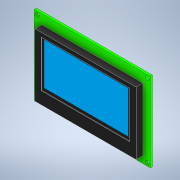
# Autodesk Inventor part: Adafruit_2675
Saved by Autodesk Inventor 2021 (Build 250183000, 183)
## iProperties
Created: 2020-11-05
Part Number: Adafruit_2675
Material: Generic
Document SubType Name: Modeling
Designer: Viktor
Density: 1 g/cm^3
Appearance: Default
Author: Viktor
Autodesk Inventor part; units mm, degrees
ref_plane "YZ Plane" through (0, 0, 0) normal (1, 0, 0) x (0, 1, 0)
ref_plane "XZ Plane" through (0, 0, 0) normal (0, 1, 0) x (-1, 0, 0)
ref_plane "XY Plane" through (0, 0, 0) normal (0, 0, 1) x (1, 0, 0)
sketch "Sketch1" plane through (0, 0, 0) normal (0, 0, 1) x (1, 0, 0)
  line L0 (-42.5, -29) -> (42.5, -29)
  line L1 (42.5, -29) -> (42.5, 29)
  line L2 (42.5, 29) -> (-42.5, 29)
  line L3 (-42.5, 29) -> (-42.5, -29)
  line L4 (-42.5, -29) -> (42.5, 29) construction
  line L5 (42.5, -29) -> (-42.5, 29) construction
  point P0 (0, 0)
  dimension "d0" = 85
  dimension "d1" = 58
  constraints: 12 end point, 2 midpoint, 2 parallel, 1 horizontal, 1 perpendicular
  measures "d0" distance of L1.end L2.end
  measures "d1" distance of L0.end L1.end
extrude "Extrusion1" add sketch "Sketch1" along normal blind 1.6
sketch "Sketch2" plane through (0, 0, 1.6) normal (0, 0, 1) x (1, 0, 0)
  line L0 (-59.5, 0) -> (59.5, 0) construction
  line L1 (0, -40.6) -> (0, 40.6) construction
  circle A0 centre (-40.3, 26.8) radius 1.6
  line L2 (42.5, 29) -> (-42.5, 29) construction
  line L3 (-42.5, 29) -> (-42.5, -29) construction
  circle A1 centre (40.3, 26.8) radius 1.6
  circle A2 centre (-40.3, -26.8) radius 1.6
  line L4 (42.5, -29) -> (-42.5, -29) construction
  circle A3 centre (40.3, -26.8) radius 1.6
  point P0 (0, 0)
  dimension "d4" = 3.2
  dimension "d5" = 0.6
  dimension "d6" = 0.6
  constraints: 4 centre point, 4 symmetric about line, 2 end point, 3 other
  measures "d4" diameter of A0
  measures "d5" distance edge to line of A0 L2
  measures "d6" distance edge to line of A0 L3
extrude "Extrusion2" cut sketch "Sketch2" against normal through all
sketch "Sketch3" plane through (0, 0, 1.6) normal (0, 0, 1) x (1, 0, 0)
  line L0 (0, 40.6) -> (0, -40.6) projected
  line L1 (-37, -24) -> (37, -24)
  line L2 (37, -24) -> (37, 22)
  line L3 (37, 22) -> (-37, 22)
  line L4 (-37, 22) -> (-37, -24)
  line L5 (-37, -24) -> (37, 22) construction
  line L6 (37, -24) -> (-37, 22) construction
  line L7 (-59.5, 0) -> (59.5, 0) projected
  point P0 (0, -1)
  dimension "d9" = 46
  dimension "d10" = 74
  dimension "d25" = 1
  constraints: 12 end point, 2 midpoint, 2 parallel, 1 horizontal, 1 perpendicular, 1 point on line
  measures "d9" distance of L3.end L1.start
  measures "d10" distance of L2.end L3.end
  measures "d25" distance from line of L7 point (0, -1)
extrude "Extrusion3" add sketch "Sketch3" along normal blind 5 separate body
sketch "Sketch4" plane through (0, 0, 6.6) normal (0, 0, 1) x (1, 0, 0)
  line L0 (0, -40.6) -> (0, 40.6) projected
  line L1 (-32.5, -15) -> (32.5, -15)
  line L2 (32.5, -15) -> (32.5, 19)
  line L3 (32.5, 19) -> (-32.5, 19)
  line L4 (-32.5, 19) -> (-32.5, -15)
  line L5 (-32.5, -15) -> (32.5, 19) construction
  line L6 (32.5, -15) -> (-32.5, 19) construction
  line L7 (37, 22) -> (-37, 22) projected
  point P0 (0, 0)
  point P1 (0, 2)
  dimension "d13" = 34
  dimension "d14" = 65
  dimension "d15" = 3
  constraints: 12 end point, 2 midpoint, 2 parallel, 1 horizontal, 1 perpendicular, 1 point on line
  measures "d13" distance of L3.end L1.start
  measures "d14" distance of L2.end L3.end
  measures "d15" distance between parallel lines of L7 L3
extrude "Extrusion4" cut sketch "Sketch4" against normal blind 0.5 bodies 2
sketch "Sketch5" plane through (0, 0, 6.1) normal (0, 0, 1) x (1, 0, 0)
  line L0 (0, 40.6) -> (0, -40.6) projected
  line L1 (-30.705, -12.69) -> (30.705, -12.69)
  line L2 (30.705, -12.69) -> (30.705, 18)
  line L3 (30.705, 18) -> (-30.705, 18)
  line L4 (-30.705, 18) -> (-30.705, -12.69)
  line L5 (-30.705, -12.69) -> (30.705, 18) construction
  line L6 (30.705, -12.69) -> (-30.705, 18) construction
  line L7 (37, 22) -> (-37, 22) projected
  point P0 (0, 0)
  point P1 (0, 2.655)
  dimension "d18" = 30.69
  dimension "d19" = 61.41
  dimension "d20" = 4
  constraints: 12 end point, 2 midpoint, 2 parallel, 1 horizontal, 1 perpendicular, 1 point on line
  measures "d18" distance of L3.end L1.start
  measures "d19" distance of L2.end L3.end
  measures "d20" distance between parallel lines of L7 L3
extrude "Extrusion5" cut sketch "Sketch5" against normal blind 0.5 bodies 2
sketch "Sketch6" plane through (0, 0, 5.6) normal (0, 0, 1) x (1, 0, 0)
  line L0 (30.705, -12.69) -> (-30.705, -12.69) projected
  line L1 (30.705, 18) -> (30.705, -12.69) projected
  line L2 (-30.705, 18) -> (30.705, 18) projected
  line L3 (-30.705, -12.69) -> (-30.705, 18) projected
  point P0 (0, 0)
extrude "Extrusion6" add sketch "Sketch6" along normal blind 0.5 separate body
sketch "Sketch7" plane through (0, 0, 6.6) normal (0, 0, 1) x (1, 0, 0)
  circle A0 centre (0, 0) radius 6.7082
  constraints: 1 centre point, 1 coincident
equation "\"d6\" = d5"
body "Solid1"
body "Solid2"
body "Solid3"
